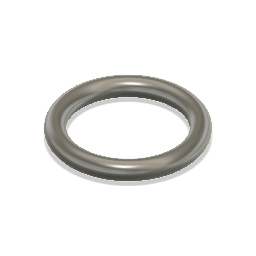
Peg_Ring (Autodesk Fusion 360 design; units mm, degrees)
Autodesk Fusion 360 part; units mm, degrees
sketch "Sketch1" plane through (0, 0, 0) normal (0, 1, 0) x (1, 0, 0)
  circle A0 centre (0, 0) radius 4.35
  circle A1 centre (0, 0) radius 5.35
  dimension "d1" = 8.7
  dimension "d2" = 10.7
  constraint coincident A0.centre A1.centre
  constraint concentric A0 A1
  measures "d1" diameter of A0
  measures "d2" diameter of A1
extrude "Extrude1" [suppressed]
torus "TorusPrimitive1" add centre line diameter 10.7 section diameter 1.7 placed x (1, 0, 0) y (0, 0, -1) z (0, 1, 0) at (0, 0, 0)
